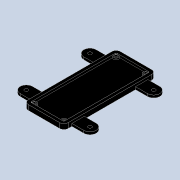
# Autodesk Inventor part: Elegoo 8 Channel Relay Module
Saved by Autodesk Inventor 2022 (Build 260153000, 153)
## iProperties
Created: 2022-01-02
Part Number: Elegoo 8 Channel Relay Module
Material: Generic
Document SubType Name: Modeling
Designer: Coy
Density: 1 g/cm^3
Appearance: Anodized - Black
Author: Coy
Autodesk Inventor part; units mm, degrees
ref_plane "YZ Plane" through (0, 0, 0) normal (1, 0, 0) x (0, 1, 0)
ref_plane "XZ Plane" through (0, 0, 0) normal (0, 1, 0) x (-1, 0, 0)
ref_plane "XY Plane" through (0, 0, 0) normal (0, 0, 1) x (1, 0, 0)
sketch "Sketch1" plane through (0, 0, 0) normal (0, 1, 0) x (-1, 0, 0)
  line L0 (1.5, 0) -> (51, 0)
  line L1 (52.5, 1.5) -> (52.5, 133)
  line L2 (51, 134.5) -> (1.5, 134.5)
  line L3 (0, 133) -> (0, 1.5)
  arc A0 (52.5, 133) -> (51, 134.5) centre (51, 133) ccw
  arc A1 (51, 0) -> (52.5, 1.5) centre (51, 1.5) ccw
  arc A2 (0, 1.5) -> (1.5, 0) centre (1.5, 1.5) ccw
  arc A3 (1.5, 134.5) -> (0, 133) centre (1.5, 133) ccw
  line L4 (57.5, 133) -> (57.5, 1.5)
  arc A4 (51, -5) -> (57.5, 1.5) centre (51, 1.5) ccw
  line L5 (51, -5) -> (1.5, -5)
  arc A5 (-5, 1.5) -> (1.5, -5) centre (1.5, 1.5) ccw
  line L6 (-5, 1.5) -> (-5, 133)
  arc A6 (1.5, 139.5) -> (-5, 133) centre (1.5, 133) ccw
  line L7 (1.5, 139.5) -> (51, 139.5)
  arc A7 (57.5, 133) -> (51, 139.5) centre (51, 133) ccw
  point P0 (0, 0)
  point P1 (52.5, 134.5)
  point P2 (52.5, 0)
  point P3 (0, 134.5)
  dimension "d0" = 52.5
  dimension "d1" = 134.5
  dimension "d2" = 1.5
  dimension "d3" = 5
  constraints: 16 end point, 16 point on circle, 8 centre point, 8 point on line, 8 tangent, 4 parallel, 3 equal radius, 2 perpendicular, 1 horizontal, 7 other
  measures "d0" distance of point (0, 134.5) point (52.5, 134.5)
  measures "d1" distance of point (52.5, 134.5) point (52.5, 0)
  measures "d2" radius of A0
  measures "d3" distance between parallel lines of L1 L4
extrude "Extrusion1" add sketch "Sketch1" against normal blind 4
sketch "Sketch2" plane through (0, -4, 0) normal (0, -1, 0) x (1, 0, 0)
  line L0 (5, 1.5) -> (5, 133) projected
  arc A0 (5, 133) -> (-1.5, 139.5) centre (-1.5, 133) ccw projected
  line L1 (-1.5, 139.5) -> (-51, 139.5) projected
  arc A1 (-51, 139.5) -> (-57.5, 133) centre (-51, 133) ccw projected
  line L2 (-57.5, 133) -> (-57.5, 1.5) projected
  arc A2 (-57.5, 1.5) -> (-51, -5) centre (-51, 1.5) ccw projected
  line L3 (-51, -5) -> (-1.5, -5) projected
  arc A3 (-1.5, -5) -> (5, 1.5) centre (-1.5, 1.5) ccw projected
  arc A4 (-1.5, 0) -> (0, 1.5) centre (-1.5, 1.5) ccw projected
  line L4 (-1.5, 0) -> (-51, 0) projected
  arc A5 (-52.5, 1.5) -> (-51, 0) centre (-51, 1.5) ccw projected
  line L5 (-52.5, 1.5) -> (-52.5, 133) projected
  arc A6 (-51, 134.5) -> (-52.5, 133) centre (-51, 133) ccw projected
  line L6 (-51, 134.5) -> (-1.5, 134.5) projected
  arc A7 (0, 133) -> (-1.5, 134.5) centre (-1.5, 133) ccw projected
  line L7 (0, 133) -> (0, 1.5) projected
  line L8 (23.75, 117.25) -> (-76.25, 117.25) construction
  line L9 (-76.25, 117.25) -> (-76.25, 17.25) construction
  line L10 (-76.25, 17.25) -> (23.75, 17.25) construction
  line L11 (23.75, 17.25) -> (23.75, 117.25) construction
  circle A8 centre (23.75, 117.25) radius 2.75
  arc A9 (23.75, 107.5) -> (23.75, 127) centre (23.75, 117.25) ccw
  line L12 (5, 1.5) -> (5, 133) projected
  line L13 (5, 127) -> (23.75, 127)
  line L14 (5, 107.5) -> (23.75, 107.5)
  line L15 (23.75, 67.25) -> (-76.25, 67.25) construction
  line L16 (-26.25, 67.25) -> (-26.25, 117.25) construction
  circle A10 centre (23.75, 17.25) radius 2.75
  arc A11 (23.75, 7.5) -> (23.75, 27) centre (23.75, 17.25) ccw
  line L17 (5, 7.5) -> (23.75, 7.5)
  line L18 (5, 27) -> (23.75, 27)
  circle A12 centre (-76.25, 117.25) radius 2.75
  arc A13 (-76.25, 127) -> (-76.25, 107.5) centre (-76.25, 117.25) ccw
  line L19 (-57.5, 127) -> (-76.25, 127)
  line L20 (-57.5, 107.5) -> (-76.25, 107.5)
  arc A14 (-76.25, 27) -> (-76.25, 7.5) centre (-76.25, 17.25) ccw
  circle A15 centre (-76.25, 17.25) radius 2.75
  line L21 (-57.5, 7.5) -> (-76.25, 7.5)
  line L22 (-57.5, 27) -> (-76.25, 27)
  point P0 (0, 0)
  dimension "d6" = 100
  dimension "d7" = 100
  dimension "d8" = 62.5
  dimension "d9" = 144.5
  dimension "d10" = 18.75
  dimension "d11" = 22.25
  dimension "d12" = 5.5
  dimension "d13" = 7
  constraints: 28 end point, 15 symmetric about line, 8 centre point, 8 point on circle, 4 midpoint, 3 perpendicular, 3 point on line, 2 parallel, 2 tangent, 1 coincident, 1 horizontal, 6 other
  measures "d6" distance of L10.end L9.end
  measures "d7" distance of L9.end L8.end
  measures "d8" distance between parallel lines of L2 L0
  measures "d9" distance between parallel lines of L3 L1
  measures "d10" distance between parallel lines of L0 L11
  measures "d11" distance between parallel lines of L1 L8
  measures "d12" diameter of A8
  measures "d13" radial gap between concentric circles of A8 A9
extrude "Extrusion2" add sketch "Sketch2" along normal blind 4 contours A3 L3 A2 L2 A1 L1 A0 L0 | L0 L18 A11 L17 | L0 L13 A9 L14 | L21 A14 L22 L2 | L20 A13 L19 L2 | L4 A5 L5 A6 L6 A7 L7 A4
sketch "Sketch3" plane through (0, -4, 0) normal (0, 1, 0) x (1, 0, 0)
  line L0 (-49.575, -131.425) -> (-2.925, -131.425) construction
  line L1 (-2.925, -131.425) -> (-2.925, -3.075) construction
  line L2 (-2.925, -3.075) -> (-49.575, -3.075) construction
  line L3 (-49.575, -3.075) -> (-49.575, -131.425) construction
  line L4 (-49.575, -131.425) -> (-49.575, -134.5) construction
  line L5 (-1.5, -134.5) -> (-51, -134.5) construction
  line L6 (-49.575, -131.425) -> (-52.5, -131.425) construction
  line L7 (-52.5, -1.5) -> (-52.5, -133) construction
  line L8 (-2.925, -3.075) -> (0, -3.075) construction
  line L9 (0, -1.5) -> (0, -133) construction
  line L10 (-2.925, -3.075) -> (-2.925, 0) construction
  line L11 (-51, 0) -> (-1.5, 0) construction
  circle A0 centre (-49.575, -131.425) radius 4
  circle A1 centre (-2.925, -131.425) radius 4
  circle A2 centre (-2.925, -3.075) radius 4
  circle A3 centre (-49.575, -3.075) radius 4
  point P0 (0, 0)
  dimension "d16" = 46.65
  dimension "d17" = 128.35
  dimension "d18" = 8
  dimension "d19" = 8
  dimension "d20" = 8
  dimension "d21" = 8
  constraints: 16 end point, 5 parallel, 4 centre point, 4 coincident, 4 point on line, 3 perpendicular, 1 horizontal, 1 vertical
  measures "d16" distance of L2.end L1.end
  measures "d17" distance of L1.end L0.end
  measures "d18" diameter of A0
  measures "d19" diameter of A1
  measures "d20" diameter of A2
  measures "d21" diameter of A3
extrude "Extrusion3" add sketch "Sketch3" along normal blind 2.4
sketch "Sketch4" plane through (0, -1.6, 0) normal (0, 1, 0) x (1, 0, 0)
  line L0 (-47.0168, -134.5) -> (-51, -134.5) projected
  arc A0 (-47.0168, -134.5) -> (-52.5, -128.6966) centre (-49.575, -131.425) ccw projected
  line L1 (-52.5, -133) -> (-52.5, -128.6966) projected
  arc A1 (-52.5, -133) -> (-51, -134.5) centre (-51, -133) ccw projected
  line L2 (0, -128.6966) -> (0, -133) projected
  arc A2 (0, -128.6966) -> (-5.4832, -134.5) centre (-2.925, -131.425) ccw projected
  line L3 (-1.5, -134.5) -> (-5.4832, -134.5) projected
  arc A3 (-1.5, -134.5) -> (0, -133) centre (-1.5, -133) ccw projected
  line L4 (-52.5, -5.8034) -> (-52.5, -1.5) projected
  arc A4 (-52.5, -5.8034) -> (-47.0168, 0) centre (-49.575, -3.075) ccw projected
  line L5 (-51, 0) -> (-47.0168, 0) projected
  arc A5 (-51, 0) -> (-52.5, -1.5) centre (-51, -1.5) ccw projected
  line L6 (-5.4832, 0) -> (-1.5, 0) projected
  arc A6 (-5.4832, 0) -> (0, -5.8034) centre (-2.925, -3.075) ccw projected
  line L7 (0, -1.5) -> (0, -5.8034) projected
  arc A7 (0, -1.5) -> (-1.5, 0) centre (-1.5, -1.5) ccw projected
  circle A8 centre (-49.575, -131.425) radius 1.5
  arc A9 (-52.5, -5.8034) -> (-47.0168, 0) centre (-49.575, -3.075) ccw projected
  circle A10 centre (-49.575, -3.075) radius 1.5
  circle A11 centre (-2.925, -3.075) radius 1.5
  arc A12 (0, -128.6966) -> (-5.4832, -134.5) centre (-2.925, -131.425) ccw projected
  circle A13 centre (-2.925, -131.425) radius 1.5
  point P0 (0, 0)
  dimension "d24" = 3
  dimension "d25" = 3
  dimension "d26" = 3
  dimension "d27" = 3
  constraints: 4 centre point, 4 coincident
  measures "d24" diameter of A8
  measures "d25" diameter of A13
  measures "d26" diameter of A10
  measures "d27" diameter of A11
extrude "Extrusion4" cut sketch "Sketch4" against normal through all contours A8 | A10 | A11 | A13
chamfer "Chamfer1" distance 1 angle 45 4 edges at (-51.075, -1.6, 131.425) (-4.425, -1.6, 131.425) (-4.425, -1.6, 3.075) (-51.075, -1.6, 3.075)
equation "\"d10\" = -0.5 * d8 + 0.5 * d6"
equation "\"d11\" = -0.5 * d7 + 0.5 * d9"
equation "\"d19\" = d18"
equation "\"d20\" = d18"
equation "\"d21\" = d18"
equation "\"d25\" = d24"
equation "\"d26\" = d24"
equation "\"d27\" = d24"
body "Solid1"
